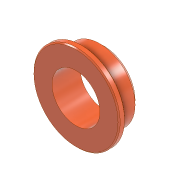
# Autodesk Inventor part: Print_Parts_P
Saved by Autodesk Inventor 2020.1 (Build 241239000, 239)
## iProperties
Created: 2020-10-05
Part Number: Print_Parts_P
Material: PC/ABS プラスチック
Document SubType Name: Modeling
Designer: kenta iguchi
Density: 0.357273 g/cm^3
Appearance: 滑らか - 淡いオレンジ
Author: kenta iguchi
Autodesk Inventor part; units mm, degrees
ref_plane "YZ Plane" through (0, 0, 0) normal (1, 0, 0) x (0, 1, 0)
ref_plane "XZ Plane" through (0, 0, 0) normal (0, 1, 0) x (-1, 0, 0)
ref_plane "XY Plane" through (0, 0, 0) normal (0, 0, 1) x (1, 0, 0)
sketch "スケッチ1" plane through (0, 0, 0) normal (0, 0, 1) x (1, 0, 0)
  circle A0 centre (0, 0) radius 16.4
  dimension "d0" = 32.8
  constraints: 1 centre point, 1 coincident
  measures "d0" diameter of A0
extrude "押し出し1" add sketch "スケッチ1" along normal blind 10
sketch "スケッチ2" plane through (0, 0, 10) normal (0, 0, 1) x (1, 0, 0)
  circle A0 centre (0, 0) radius 16.4 projected
  circle A1 centre (0, 0) radius 20
  dimension "d3" = 40
  constraints: 1 centre point, 1 coincident
  measures "d3" diameter of A1
extrude "押し出し2" add sketch "スケッチ2" along normal blind 3 contours A0 | A1
chamfer "面取り1" distance 2 angle 45 1 edges at (-16.4, 0, 0)
chamfer "面取り2" distance 0.5 angle 45 2 edges at (-20, 0, 13) (-20, 0, 10)
sketch "スケッチ3" plane through (0, 0, 13) normal (0, 0, 1) x (1, 0, 0)
  circle A0 centre (0, 0) radius 19.5 projected
  circle A1 centre (0, 0) radius 11.1
  dimension "d12" = 22.2
  constraints: 1 centre point, 1 coincident
  measures "d12" diameter of A1
extrude "押し出し3" cut sketch "スケッチ3" against normal through all contours A1
